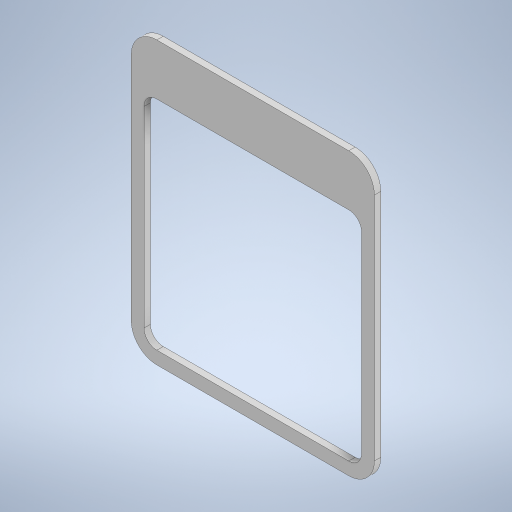
# Autodesk Inventor part: frame_outer
Saved by Autodesk Inventor 2023 (Build 270158000, 158)
## iProperties
Created: 2022-11-05
Part Number: frame_outer
Material: Generisch
Document SubType Name: Modeling
Designer: RubenStein
Density: 1 g/cm^3
Appearance: Vorgabe
Author: RubenStein
Autodesk Inventor part; units mm, degrees
ref_plane "YZ Plane" through (0, 0, 0) normal (1, 0, 0) x (0, 1, 0)
ref_plane "XZ Plane" through (0, 0, 0) normal (0, 1, 0) x (-1, 0, 0)
ref_plane "XY Plane" through (0, 0, 0) normal (0, 0, 1) x (1, 0, 0)
sketch "Skizze1" plane through (0, 0, 0) normal (0, 0, 1) x (1, 0, 0)
  line L0 (0, 0) -> (190, 0)
  line L1 (190, 0) -> (190, 220)
  line L2 (190, 220) -> (0, 220)
  line L3 (0, 220) -> (0, 0)
  line L4 (10, 10) -> (180, 10)
  line L5 (180, 10) -> (180, 180)
  line L6 (180, 180) -> (10, 180)
  line L7 (10, 180) -> (10, 10)
  dimension "d0" = 170
  dimension "d1" = 190
  dimension "d2" = 10
  dimension "d3" = 10
  dimension "d8" = 220
  constraints: 16 end point, 4 parallel, 3 perpendicular, 2 horizontal
  measures "d0" distance of L5.end L6.end
  measures "d1" distance of L1.end L2.end
  measures "d2" distance between parallel lines of L3 L7
  measures "d3" distance between parallel lines of L0 L4
  measures "d8" distance of L0.end L1.end
extrude "Extrusion1" add sketch "Skizze1" along normal blind 5
fillet "Rundung1" radius 10 4 edges at (10, 180, 2.5) (180, 180, 2.5) (180, 10, 2.5) (10, 10, 2.5)
fillet "Rundung2" radius 20 4 edges at (190, 0, 2.5) (190, 220, 2.5) (0, 220, 2.5) (0, 0, 2.5)
equation "\"d3\" = d2"
